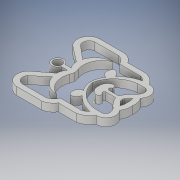
# Autodesk Inventor part: kylo_v2
Saved by Autodesk Inventor 2019 (Build 230136000, 136)
## iProperties
Created: 2019-10-18
Part Number: kylo_v2
Material: Generic
Document SubType Name: Modeling
Designer: ADK
Density: 1 g/cm^3
Appearance: Default
Author: ADK
Autodesk Inventor part; units mm, degrees
note: some values were not read from the file. Chosen so that the rebuilt part matches the saved one: second side of "Extrusion2".
ref_plane "YZ Plane" through (0, 0, 0) normal (1, 0, 0) x (0, 1, 0)
ref_plane "XZ Plane" through (0, 0, 0) normal (0, 1, 0) x (-1, 0, 0)
ref_plane "XY Plane" through (0, 0, 0) normal (0, 0, 1) x (1, 0, 0)
sketch "Sketch1" plane through (0, 0, 0) normal (0, 1, 0) x (-1, 0, 0)
  line L0 (-30, 30) -> (30, 30)
  line L1 (30, 30) -> (30, -30)
  line L2 (30, -30) -> (-30, -30)
  line L3 (-30, -30) -> (-30, 30)
  line L4 (-30, 30) -> (30, -30) construction
  line L5 (30, 30) -> (-30, -30) construction
  point P0 (0, 0)
  dimension "d0" = 60
  dimension "d1" = 60
  constraints: 12 end point, 2 midpoint, 2 parallel, 1 horizontal, 1 perpendicular
  measures "d0" distance of L1.end L2.end
  measures "d1" distance of L0.end L1.end
extrude "Extrusion1" add sketch "Sketch1" along normal blind 3
sketch "Sketch2" plane through (0, 3, 0) normal (0, 1, 0) x (1, 0, 0)
  line L0 (-14.2568, -16.0971) -> (-4.4072, -16.0971)
  arc A0 (-4.4072, -16.0971) -> (-0.6208, -13.5234) centre (-5.3347, -10.6606) ccw
  line L1 (-0.6208, -13.5234) -> (6.3792, -13.5234)
  arc A1 (6.3792, -13.5234) -> (10.8868, -10.3804) centre (4.8197, -6.4828) ccw
  arc A2 (10.8868, -10.3804) -> (13.7823, -4.144) centre (11.0028, -6.6439) ccw
  arc A3 (13.7823, -4.144) -> (14.6979, -0.0584) centre (8.4389, -0.8011) ccw
  arc A4 (-17.1476, -8.6988) -> (-14.2568, -16.0971) centre (-13.9489, -11.7129) ccw
  line L2 (-17.1476, -8.6988) -> (-10.8795, -3.8506)
  arc A5 (-9.8562, -0.8011) -> (-10.9349, -3.8935) centre (-5.1826, -4.1657) ccw
  line L3 (-9.8562, -0.8011) -> (-9.8562, -0.0584)
  line L4 (-14.0136, -14.1392) -> (-4.7951, -14.1392)
  arc A6 (-15.847, -10.3804) -> (-14.0136, -14.1392) centre (-13.7788, -11.6982) ccw
  line L5 (-15.847, -10.3804) -> (-10.5225, -5.8935)
  arc A7 (-10.5225, -5.8935) -> (-3.852, -10.9628) centre (-3.7142, -3.8582) ccw
  arc A8 (-8.0837, -1.6881) -> (-3.852, -10.9628) centre (-1.2019, -4.151) ccw
  arc A9 (-8.0837, -1.6881) -> (-7.6688, -0.0584) centre (-13.0672, 0.4482) ccw
  arc A10 (-4.7951, -14.1392) -> (-1.782, -11.521) centre (-5.6993, -10.0558) ccw
  line L6 (-1.782, -11.521) -> (6.1413, -11.521)
  arc A11 (6.1413, -11.521) -> (8.3233, -10.2779) centre (5.8175, -8.4161) ccw
  arc A12 (1.5968, -6.4828) -> (8.3233, -10.2779) centre (10.6825, 1.7625) ccw
  arc A13 (-0.8314, -8.6988) -> (1.5968, -6.4828) centre (-1.5815, -5.4386) ccw
  arc A14 (0.0663, -4.3882) -> (-0.8314, -8.6988) centre (0.5503, -6.7378) ccw
  arc A15 (-1.4509, -0.0584) -> (0.0663, -4.3882) centre (5.0784, -0.2012) ccw
  arc A16 (-0.8314, -0.0584) -> (8.4389, -8.4161) centre (9.3519, 1.9167) ccw
  line L7 (8.4389, -8.4161) -> (11.2507, -8.4161)
  arc A17 (11.2507, -8.4161) -> (12.6649, -6.8375) centre (11.0079, -6.7758) ccw
  arc A18 (12.6649, -6.8375) -> (11.0955, -4.0646) centre (9.1189, -7.0139) ccw
  arc A19 (8.6889, -0.6246) -> (11.0955, -4.0646) centre (18.4614, 3.6503) ccw
  line L8 (8.6889, -0.6246) -> (4.9462, -0.6246)
  arc A20 (4.9462, -0.6246) -> (4.9462, -1.9862) centre (5.0451, -1.3054) ccw
  arc A21 (1.5441, -0.0584) -> (3.7899, -3.4449) centre (4.5437, -0.5071) ccw
  arc A22 (3.7899, -3.4449) -> (4.9462, -1.9862) centre (3.9013, -2.3455) ccw
  arc A23 (12.2833, -2.5577) -> (12.6649, -0.0584) centre (8.2588, -0.6644) ccw
  line L9 (12.2956, -2.5313) -> (10.7711, -0.7223)
  arc A24 (10.6825, -0.0584) -> (10.7711, -0.7223) centre (12.2958, -0.1811) ccw
  line L10 (-14.2568, 15.9802) -> (-4.4072, 15.9802)
  arc A25 (-0.6208, 13.4065) -> (-4.4072, 15.9802) centre (-5.3347, 10.5438) ccw
  line L11 (-0.6208, 13.4065) -> (6.3792, 13.4065)
  arc A26 (10.8868, 10.2636) -> (6.3792, 13.4065) centre (4.8197, 6.3659) ccw
  arc A27 (13.7823, 4.0272) -> (10.8868, 10.2636) centre (11.0028, 6.5271) ccw
  arc A28 (14.6979, -0.0584) -> (13.7823, 4.0272) centre (8.4389, 0.6842) ccw
  arc A29 (-14.2568, 15.9802) -> (-17.1476, 8.582) centre (-13.9489, 11.596) ccw
  line L12 (-17.1476, 8.582) -> (-10.8795, 3.7338)
  arc A30 (-10.9349, 3.7766) -> (-9.8562, 0.6842) centre (-5.1826, 4.0488) ccw
  line L13 (-9.8562, 0.6842) -> (-9.8562, -0.0584)
  line L14 (-14.0136, 14.0224) -> (-4.7951, 14.0224)
  arc A31 (-14.0136, 14.0224) -> (-15.847, 10.2636) centre (-13.7788, 11.5813) ccw
  line L15 (-15.847, 10.2636) -> (-10.5225, 5.7766)
  arc A32 (-3.852, 10.8459) -> (-10.5225, 5.7766) centre (-3.7142, 3.7413) ccw
  arc A33 (-3.852, 10.8459) -> (-8.0837, 1.5713) centre (-1.2019, 4.0341) ccw
  arc A34 (-7.6688, -0.0584) -> (-8.0837, 1.5713) centre (-13.0672, -0.565) ccw
  arc A35 (-1.782, 11.4041) -> (-4.7951, 14.0224) centre (-5.6993, 9.9389) ccw
  line L16 (-1.782, 11.4041) -> (6.1413, 11.4041)
  arc A36 (8.3233, 10.161) -> (6.1413, 11.4041) centre (5.8175, 8.2992) ccw
  arc A37 (8.3233, 10.161) -> (1.5968, 6.3659) centre (10.6825, -1.8794) ccw
  arc A38 (1.5968, 6.3659) -> (-0.8314, 8.582) centre (-1.5815, 5.3218) ccw
  arc A39 (-0.8314, 8.582) -> (0.0663, 4.2713) centre (0.5503, 6.6209) ccw
  arc A40 (0.0663, 4.2713) -> (-1.4509, -0.0584) centre (5.0784, 0.0844) ccw
  arc A41 (8.4389, 8.2992) -> (-0.8314, -0.0584) centre (9.3519, -2.0336) ccw
  line L17 (8.4389, 8.2992) -> (11.2507, 8.2992)
  arc A42 (12.6649, 6.7206) -> (11.2507, 8.2992) centre (11.0079, 6.659) ccw
  arc A43 (11.0955, 3.9478) -> (12.6649, 6.7206) centre (9.1189, 6.8971) ccw
  arc A44 (11.0955, 3.9478) -> (8.6889, 0.5078) centre (18.4614, -3.7672) ccw
  line L18 (8.6889, 0.5078) -> (4.9462, 0.5078)
  arc A45 (4.9462, 1.8694) -> (4.9462, 0.5078) centre (5.0451, 1.1886) ccw
  arc A46 (3.7899, 3.328) -> (1.5441, -0.0584) centre (4.5437, 0.3902) ccw
  arc A47 (4.9462, 1.8694) -> (3.7899, 3.328) centre (3.9013, 2.2286) ccw
  arc A48 (12.6649, -0.0584) -> (12.2833, 2.4409) centre (8.2588, 0.5476) ccw
  line L19 (12.2956, 2.4145) -> (10.7711, 0.6055)
  arc A49 (10.7711, 0.6055) -> (10.6825, -0.0584) centre (12.2958, 0.0642) ccw
  point P0 (0, 0)
  point P1 (0, -0.1169)
  dimension "d23" = 7
  constraints: 106 point on circle, 50 centre point, 40 end point, 6 horizontal, 2 point on line
  measures "d23" distance of L1.start L1.end
extrude "Extrusion2" add sketch "Sketch2" along normal blind 3
sketch "Sketch3" plane through (0, 0, 0) normal (0, -1, 0) x (1, 0, 0)
  circle A0 centre (0, 0) radius 25
  line L0 (-30, 30) -> (30, 30) projected
  line L1 (-30, -30) -> (30, -30)
  line L2 (30, -30) -> (30, 30)
  line L3 (30, 30) -> (-30, 30)
  line L4 (-30, 30) -> (-30, -30)
  line L5 (-30, -30) -> (30, 30) construction
  line L6 (30, -30) -> (-30, 30) construction
  dimension "d33" = 50
  constraints: 12 end point, 2 midpoint, 2 parallel, 1 centre point, 1 coincident, 1 horizontal, 1 perpendicular
  measures "d33" diameter of A0
extrude "Extrusion3" cut sketch "Sketch3" against normal blind 3
sketch "Sketch4" plane through (0, 3, 0) normal (0, 1, 0) x (1, 0, 0)
  circle A0 centre (-20, 4) radius 1
  circle A1 centre (-20, -4) radius 1
  point P0 (0, 0)
  dimension "d36" = 2
  constraints: 2 centre point
  measures "d36" diameter of A0
extrude "Extrusion4" cut sketch "Sketch4" against normal blind 3
sketch "Sketch5" plane through (0, 0, 0) normal (0, 0, 1) x (1, 0, 0)
  line L0 (25.8254, 0) -> (-27.9469, 0)
  line L1 (-27.9469, 0) -> (-27.9469, 3)
  line L2 (-27.9469, 3) -> (25.8254, 3)
  line L3 (25.8254, 3) -> (25.8254, 0)
  point P0 (0, 0)
  constraints: 8 end point, 2 parallel, 1 horizontal, 1 perpendicular
extrude "Extrusion5" cut sketch "Sketch5" along normal blind 32.5 and the other way blind 29
sketch "Sketch6" plane through (-9.8562, 6, -0.6842) normal (-1, 0, 0) x (0, 0, 1)
  line L0 (1.4853, -3) -> (0, -3) projected
  line L1 (4.5777, 0) -> (1.4853, 0) projected
  line L2 (0, -3) -> (1.4853, -3)
  line L3 (1.4853, -3) -> (1.4853, 0)
  line L4 (1.4853, 0) -> (0, 0)
  line L5 (0, 0) -> (0, -3)
  point P0 (0.6842, -6)
  constraints: 8 end point, 2 parallel, 1 horizontal, 1 perpendicular
extrude "Extrusion6" add sketch "Sketch6" along normal blind 3
sketch "Sketch7" plane through (0, 0, 0) normal (0, 1, 0) x (-1, 0, 0)
  point P0 (0, 0)
sketch "Sketch8" plane through (0, 6, 0) normal (0, 1, 0) x (1, 0, 0)
  line L0 (-12.8562, -0.8011) -> (-12.8562, 0.6842) projected
  line L1 (-9.8562, 0.6842) -> (-12.8562, 0.6842) projected
  line L2 (-12.8562, -0.8011) -> (-12.8562, 0.6842)
  line L3 (-12.8562, -0.0584) -> (-14.3897, -0.0584)
  circle A0 centre (-14.3095, -0.0584) radius 1.6321
  circle A1 centre (-14.3095, -0.0584) radius 2.25
  point P0 (0, 0)
  dimension "d45" = 4.5
  constraints: 4 end point, 1 centre point, 1 coincident, 1 horizontal, 1 midpoint, 1 perpendicular, 1 point on line, 3 other
  measures "d45" diameter of A1
extrude "Extrusion7" add sketch "Sketch8" against normal blind 3
sketch "Sketch9" plane through (0, 6, 0) normal (0, 1, 0) x (1, 0, 0)
  arc A0 (-12.8562, 0.6842) -> (-12.8562, -0.8011) centre (-14.3095, -0.0584) ccw projected
  circle A1 centre (-14.3095, -0.0584) radius 1.6321
  point P0 (0, 0)
  constraints: 1 centre point, 1 coincident
extrude "Extrusion8" cut sketch "Sketch9" against normal blind 3
body "Solid1"
